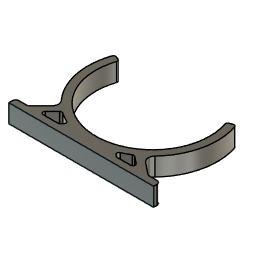
Anstandsklemme v2 (Autodesk Fusion 360 design; units mm, degrees)
Autodesk Fusion 360 part; units mm, degrees
sketch "Skizze1" plane through (0, 0, 0) normal (0, 0, 1) x (1, 0, 0)
  line L0 (0, 80) -> (0, -42.0959) construction
  line L1 (-31.8813, 0) -> (31.8813, 0)
  line L2 (31.8813, 0) -> (31.8813, 3)
  line L3 (-31.8813, 3) -> (-31.8813, 0)
  line L4 (-26.4649, 3) -> (-19.1093, 10.3556)
  line L5 (26.4649, 3) -> (18.216, 9.5813)
  line L6 (-42, 31.5) -> (42, 31.5) construction
  arc A0 (-23.5276, 40.3158) -> (23.5276, 40.3158) centre (0, 31.5) ccw
  line L7 (23.5276, 40.3158) -> (26.688, 41.5)
  line L8 (-23.5276, 40.3158) -> (-26.688, 41.5)
  arc A1 (18.216, 9.5813) -> (26.688, 41.5) centre (0, 31.5) ccw
  arc A2 (-26.688, 41.5) -> (-19.1093, 10.3556) centre (0, 31.5) ccw
  line L9 (-23.5276, 40.3158) -> (0, 31.5) construction
  line L10 (0, 31.5) -> (23.5276, 40.3158) construction
  line L11 (31.8813, 3) -> (26.4649, 3)
  line L12 (-26.4649, 3) -> (-31.8813, 3)
  arc A3 (-19.1093, 10.3556) -> (18.216, 9.5813) centre (0, 31.5) ccw
  line L13 (-26.4649, 3) -> (26.4649, 3)
  dimension "d1" = 50.25
  dimension "d2" = 3
  dimension "d4" = 31.5
  dimension "d5" = 135
  dimension "d6" = 10
  constraint vertical L0
  constraint coincident L0 A0.centre
  constraint horizontal L1
  constraint vertical L2
  constraint horizontal L11
  constraint vertical L3
  constraint symmetric L0 L2 L3
  constraint coincident L4.start L11
  constraint symmetric L0 L4.start L5.start
  constraint perpendicular L0 L6
  constraint coincident A0.centre L6
  constraint symmetric L0 L6.start L6.end
  constraint concentric A0 A1
  constraint tangent A1 L11
  constraint coincident L8.end A1
  constraint concentric A1 A2
  constraint symmetric L0 L7.end L8.end
  constraint symmetric L0 A0.start A0.end
  constraint coincident A0.centre A1.centre
  constraint parallel L8 L9
  constraint coincident origin L0
  constraint collinear L11 L12
  measures "d1" diameter of A0
  measures "d2" distance of L1.start L3.start
  measures "d4" distance of A0.centre L1
  measures "d5" angle of L4 L11
  measures "d6" distance of L6 L7.end
extrude "Extrusion1" add sketch "Skizze1" along normal blind 8
fillet "Abrundung1" radius 1 4 edges at (-23.5276, 40.3158, 4) (-26.688, 41.5, 4) (26.688, 41.5, 4) (23.5276, 40.3158, 4)
sketch "Skizze2" plane through (0, 0, 8) normal (0, 0, 1) x (-1, 0, 0)
  arc A0 (-24.4461, -40.6599) -> (-23.8478, -39.4088) centre (-24.797, -39.7235) ccw
  arc A1 (23.8478, -39.4088) -> (-23.8478, -39.4088) centre (0, -31.5) ccw
  arc A2 (23.8478, -39.4088) -> (24.4461, -40.6599) centre (24.797, -39.7235) ccw
  line L0 (24.4461, -40.6599) -> (25.7346, -41.1427)
  arc A3 (25.7346, -41.1427) -> (27.034, -40.5229) centre (26.0854, -40.2063) ccw
  arc A4 (27.034, -40.5229) -> (19.1093, -10.3556) centre (0, -31.5) ccw
  line L1 (19.1093, -10.3556) -> (26.4649, -3)
  line L2 (26.4649, -3) -> (31.8813, -3)
  line L3 (31.8813, -3) -> (31.8813, 0)
  line L4 (31.8813, 0) -> (-31.8813, 0)
  line L5 (-31.8813, 0) -> (-31.8813, -3)
  line L6 (-31.8813, -3) -> (-26.4649, -3)
  line L7 (-26.4649, -3) -> (-18.216, -9.5813)
  arc A5 (-18.216, -9.5813) -> (-27.034, -40.5229) centre (0, -31.5) ccw
  arc A6 (-27.034, -40.5229) -> (-25.7346, -41.1427) centre (-26.0854, -40.2063) ccw
  line L8 (-25.7346, -41.1427) -> (-24.4461, -40.6599)
  arc A7 (23.8478, -39.4088) -> (-23.8478, -39.4088) centre (0, -31.5) ccw
  arc A8 (27.034, -40.5229) -> (19.1093, -10.3556) centre (0, -31.5) ccw
  arc A9 (-18.216, -9.5813) -> (-27.034, -40.5229) centre (0, -31.5) ccw
  line L9 (31.8813, 0) -> (-31.8813, 0)
  circle A10 centre (0, -31.5) radius 28.5
  line L10 (16.7677, -8.4546) -> (22.2223, -3)
  line L11 (-15.725, -7.7308) -> (-21.6546, -3)
  line L12 (22.2223, -3) -> (-26.4649, -3)
  line L13 (12.9109, -3) -> (10.7896, -5.1213)
  line L14 (-12.5011, -3) -> (-10.1561, -4.871)
  dimension "d13" = 3
  dimension "d14" = 3
  dimension "d15" = 3
  dimension "d16" = 3
  constraint concentric A7 A10
  constraint coincident A10 L10.start
  constraint parallel L1 L10
  constraint parallel L4 L12
  constraint coincident A10 L11.start
  constraint coincident L11.end L12
  constraint parallel L7 L11
  constraint collinear L2 L12
  constraint coincident L12 L13.start
  constraint coincident A10 L13.end
  constraint coincident L12 L14.start
  constraint coincident A10 L14.end
  constraint parallel L11 L14
  constraint parallel L10 L13
  measures "d13" distance of L13.start L13.end
  measures "d14" distance of L14.start L14.end
  measures "d15" distance of L1 L10
  measures "d16" distance of L7 L11
extrude "Extrusion2" cut sketch "Skizze2" against normal up to surface (8 mm away) contours A10 L11 L12 L14 | A10 L10 L12 L13
fillet "Abrundung2" radius 3 2 edges at (-19.1093, 10.3556, 4) (18.216, 9.5813, 4)
fillet "Abrundung3" radius 1.5 4 edges at (31.8813, 3, 4) (26.4649, 3, 4) (-26.4649, 3, 4) (-31.8813, 3, 4)
fillet "Abrundung4" radius 1 4 edges at (21.6546, 3, 4) (15.725, 7.7308, 4) (10.1561, 4.871, 4) (12.5011, 3, 4)
fillet "Abrundung5" radius 1 4 edges at (-12.9109, 3, 4) (-10.7896, 5.1213, 4) (-16.7677, 8.4546, 4) (-22.2223, 3, 4)
sketch "Skizze3" plane through (0, 0, 0) normal (0, -1, 0) x (1, 0, 0)
  line L0 (-31.8813, 0) -> (31.8813, 0)
  line L1 (31.8813, 0) -> (31.8813, 8)
  line L2 (31.8813, 8) -> (-31.8813, 8)
  line L3 (-31.8813, 8) -> (-31.8813, 0)
equation "d4 = ( 63 / 2 ) * 1 mm"
